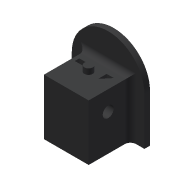
# Autodesk Inventor part: querylab
Saved by Autodesk Inventor 2022 Beta2 (Build 260130000, 130) ContinuousBuild 0
## iProperties
Shininess: 64.0
Length Units: 11269
Angle Units: 11279
Time Units: 11290
Mass Units: 11283
Length Display Precision: 3
Angle Display Precision: 2
Compacted: True
Part Number: querylab
Document SubType Name: Modeling
Created: 2004-02-27
Designer: mpaknia
Manufacturer: Standard
Standards Organization: Custom
Density: 1 g/cm^3
Material: Generic
Appearance: Generic
Density: 0.0
Volumn: 0.0
Area: 0.0
PropertySet Name: Model Information
Control State: 0
Master: False
Checked Out: False
Author: mpaknia
Autodesk Inventor part; units mm, degrees
ref_plane "YZ Plane" through (0, 0, 0) normal (1, 0, 0) x (0, 1, 0)
ref_plane "XZ Plane" through (0, 0, 0) normal (0, 1, 0) x (-1, 0, 0)
ref_plane "XY Plane" through (0, 0, 0) normal (0, 0, 1) x (1, 0, 0)
sketch "Sketch1" plane through (0, 0, 0) normal (0, 0, 1) x (1, 0, 0)
  line L0 (-19.812, 0) -> (26.416, 0) projected
  line L1 (0, 36.83) -> (0, -16.51) projected
  line L2 (-16.51, -12.7) -> (16.51, -12.7)
  line L3 (16.51, -12.7) -> (16.51, 8.89)
  arc A0 (16.51, 8.89) -> (-16.51, 8.89) centre (0, 8.89) ccw
  line L4 (-16.51, 8.89) -> (-16.51, -12.7)
  dimension "d2" = 33.02
  dimension "d3" = 8.89
  dimension "d4" = 12.7
  constraints: 6 end point, 2 point on circle, 2 tangent, 1 centre point, 1 parallel, 1 perpendicular, 1 other
  measures "d2" distance of L2.start L2.end
  measures "d3" distance from line of L0 A0.centre
  measures "d4" distance between parallel lines of L0 L2
extrude "Extrusion1" add sketch "Sketch1" along normal blind 2.54
sketch "Sketch2" plane through (0, 0, 2.54) normal (0, 0, 1) x (1, 0, 0)
  line L0 (-16.51, -12.7) -> (-16.51, 8.89) projected
  line L1 (16.51, -12.7) -> (-16.51, -12.7) projected
  line L2 (16.51, 8.89) -> (16.51, -12.7) projected
  line L3 (-10.16, -12.7) -> (-10.16, 12.7)
  line L4 (-10.16, 12.7) -> (10.16, 12.7)
  line L5 (10.16, 12.7) -> (10.16, -12.7)
  dimension "d7" = 6.35
  dimension "d8" = 6.35
  dimension "d9" = 25.4
  constraints: 6 end point, 2 perpendicular, 2 point on line, 1 parallel
  measures "d7" distance between parallel lines of L0 L3
  measures "d8" distance between parallel lines of L2 L5
  measures "d9" distance between parallel lines of L1 L4
extrude "Extrusion2" add sketch "Sketch2" along normal blind 19
sketch "Sketch3" plane through (10.16, -12.7, 21.54) normal (1, 0, 0) x (0, 0, -1)
  line L0 (0, 25.4) -> (0, 0) projected
  line L1 (19, 25.4) -> (0, 25.4) projected
  point P0 (8.89, 16.51)
  dimension "d12" = 8.89
  dimension "d13" = 8.89
  measures "d12" distance from line of L0 point (8.89, 16.51)
  measures "d13" distance from line of L1 point (8.89, 16.51)
hole "Hole1" at (10.16, 3.81, 12.65) direction (-1, 0, 0) diameter 5 end through all
fillet "Fillet1" radius 2.54 3 edges at (10.16, 0, 2.54) (0, 12.7, 2.54) (-10.16, 0, 2.54)
sketch "Sketch6" plane through (-10.16, 12.7, 21.54) normal (0, 1, 0) x (1, 0, 0)
  line L0 (0, 16.46) -> (20.32, 16.46) projected
  line L1 (20.32, 16.46) -> (20.32, 0) projected
  line L2 (13.97, 14.555) -> (13.97, 10.6635)
  line L3 (13.97, 10.6635) -> (17.2354, 14.555)
  line L4 (17.2354, 14.555) -> (13.97, 14.555)
  dimension "d22" = 6.35
  dimension "d23" = 1.905
  dimension "d24" = 40
  dimension "d25" = 5.08
  constraints: 6 end point, 1 parallel, 1 perpendicular
  measures "d22" distance between parallel lines of L1 L2
  measures "d23" distance between parallel lines of L0 L4
  measures "d24" angle of L2 L3
  measures "d25" distance of L2.end L3.end
extrude "Extrusion3" cut sketch "Sketch6" against normal blind 12.5
sketch "Sketch7" plane through (-10.16, 12.7, 21.54) normal (0, 1, 0) x (1, 0, 0)
  line L0 (0, 16.46) -> (20.32, 16.46) projected
  line L1 (0, 16.46) -> (0, 0) projected
  circle A0 centre (8.89, 11.38) radius 1.905
  dimension "d28" = 8.89
  dimension "d29" = 5.08
  dimension "d30" = 3.81
  constraints: 1 centre point
  measures "d28" distance from line of L1 A0.centre
  measures "d29" distance from line of L0 A0.centre
  measures "d30" diameter of A0
extrude "Extrusion4" add sketch "Sketch7" along normal blind 2.54
sketch "Sketch8" plane through (-10.16, 12.7, 21.54) normal (0, 1, 0) x (1, 0, 0)
  line L0 (0, 16.46) -> (20.32, 16.46) projected
  line L1 (0, 16.46) -> (0, 0) projected
  line L2 (5.08, 14.428) -> (1.651, 14.428)
  line L3 (1.651, 14.428) -> (1.651, 12.396)
  line L4 (1.651, 12.396) -> (5.08, 12.396)
  line L5 (5.08, 12.396) -> (5.08, 14.428)
  dimension "d33" = 2.032
  dimension "d34" = 1.651
  dimension "d35" = 3.429
  dimension "d36" = 2.032
  constraints: 8 end point, 2 parallel, 1 horizontal, 1 perpendicular
  measures "d33" distance between parallel lines of L0 L2
  measures "d34" distance between parallel lines of L1 L3
  measures "d35" distance of L3.end L4.end
  measures "d36" distance of L4.end L2.start
extrude "Extrusion5" cut sketch "Sketch8" against normal blind 2.54
body "Solid1"
